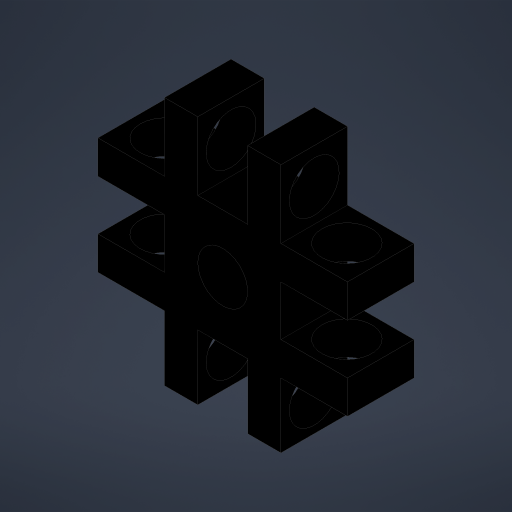
# Autodesk Inventor part: Center Connector
Saved by Autodesk Inventor 2023 (Build 270158000, 158)
## iProperties
Created: 2023-04-12
Part Number: Center Connector
Material: Generic
Document SubType Name: Modeling
Designer: vatdu
Density: 1 g/cm^3
Appearance: Default
Author: vatdu
Autodesk Inventor part; units mm, degrees
ref_plane "YZ Plane" through (0, 0, 0) normal (1, 0, 0) x (0, 1, 0)
ref_plane "XZ Plane" through (0, 0, 0) normal (0, 1, 0) x (-1, 0, 0)
ref_plane "XY Plane" through (0, 0, 0) normal (0, 0, 1) x (1, 0, 0)
sketch "Sketch1" plane through (0, 0, 0) normal (0, 0, 1) x (1, 0, 0)
  line L0 (0, 0) -> (15, 0)
  line L1 (15, 0) -> (15, 15)
  line L2 (15, 15) -> (0, 15)
  line L3 (0, 15) -> (0, 0)
  line L4 (7.5, 0) -> (7.5, 7.4)
  line L5 (7.5, 7.4) -> (6, 7.4)
  line L6 (6, 7.4) -> (6, 8.9)
  line L7 (6, 7.4) -> (7.5, 7.4) construction
  line L8 (6, 8.9) -> (9, 8.9)
  line L9 (9, 8.9) -> (9, 5.9)
  line L10 (9, 5.9) -> (6, 5.9)
  line L11 (6, 5.9) -> (6, 8.9)
  line L12 (6, 15) -> (4, 15)
  line L13 (4, 15) -> (4, 0)
  line L14 (4, 0) -> (6, 0)
  line L15 (6, 0) -> (6, 15)
  line L16 (11, 15) -> (11, 0)
  line L17 (9, 0) -> (9, 15)
  line L18 (0, 5.9) -> (15, 5.9)
  line L19 (15, 5.9) -> (15, 3.9)
  line L20 (15, 3.9) -> (0, 3.9)
  line L21 (0, 3.9) -> (0, 5.9)
  line L22 (0, 8.9) -> (15, 8.9)
  line L23 (15, 8.9) -> (15, 10.9)
  line L24 (15, 10.9) -> (0, 10.9)
  line L25 (0, 10.9) -> (0, 8.9)
  circle A0 centre (7.5, 7.4) radius 1.5
  point P0 (9, 3.9)
  point P1 (11, 3.9)
  point P2 (11, 5.9)
  point P3 (11, 8.9)
  point P4 (11, 10.9)
  point P5 (9, 10.9)
  point P6 (6, 10.9)
  point P7 (4, 10.9)
  point P8 (4, 8.9)
  point P9 (4, 5.9)
  point P10 (4, 3.9)
  point P11 (6, 3.9)
  point P12 (9, 7.4)
  point P13 (7.5, 5.9)
  point P14 (7.5, 8.9)
  dimension "d0" = 15
  dimension "d1" = 15
  dimension "d2" = 1.5
  dimension "d3" = 1.5
  dimension "d4" = 90
  dimension "d5" = 3
  dimension "d6" = 3
  dimension "d7" = 2
  dimension "d8" = 15
  dimension "d9" = 2
  dimension "d10" = 2
  constraints: 52 end point, 11 parallel, 7 perpendicular, 6 horizontal, 5 point on line, 4 symmetric about line, 1 centre point, 1 coincident, 1 midpoint, 1 vertical
  measures "d0" distance of L2.end L1.end
  measures "d1" distance of L1.end L0.end
  measures "d2" distance of L4.end L5.end
  measures "d3" distance of L5.end L6.end
  measures "d4" angle of L7 L6
  measures "d5" distance of L9.end L10.end
  measures "d6" distance of L8.end L9.end
  measures "d7" distance of L14.end L13.end
  measures "d8" distance of L19.end L20.end
  measures "d9" distance of L18.end L19.end
  measures "d10" distance of L23.end L22.end
extrude "Extrusion1" add sketch "Sketch1" along normal blind 4 contours L13 L20 L15 L0 | L3 L18 L13 L20 | L13 L18 L15 L20 | L15 L10 L4 L20 | L13 L22 L6 L11 L18 | L3 L24 L13 L22 | L17 L20 L16 L0 | L4 L10 L17 L20 | L11 A0 L10 | L13 L24 L15 L22 | L17 L18 L16 L20 | A0 L9 L10 | L6 L8 A0 | L13 L2 L15 L24 | L15 L24 L17 L8 | L16 L18 L1 L20 | L9 L22 L16 L18 | A0 L8 L9 | L17 L24 L16 L22 | L17 L2 L16 L24 | L16 L24 L1 L22
sketch "Sketch2" plane through (11, 3.9, 0) normal (0, -1, 0) x (1, 0, 0)
  line L0 (0, 0) -> (0, 4) projected
  line L1 (0, 2) -> (3.9254, 2)
  circle A0 centre (1.9627, 2) radius 1.5
  point P0 (-11, 0)
  dimension "d13" = 3
  constraints: 2 end point, 2 midpoint, 1 centre point, 1 horizontal
  measures "d13" diameter of A0
extrude "Extrusion2" cut sketch "Sketch2" against normal blind 15
pattern_circular "Circular Pattern1" count 4 over 360 about axis through (7.5, 7.4, 0) along (0, 0, 1) of "Extrusion2"
body "Solid1"
